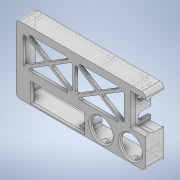
# Autodesk Inventor part: top_squr
Saved by Autodesk Inventor 2021 (Build 250183000, 183)
## iProperties
Created: 2025-01-04
Part Number: top_squr
Material: Generic
Document SubType Name: Modeling
Designer: Toby
Density: 1 g/cm^3
Appearance: Default
Author: Toby
Autodesk Inventor part; units mm, degrees
ref_plane "YZ Plane" through (0, 0, 0) normal (1, 0, 0) x (0, 1, 0)
ref_plane "XZ Plane" through (0, 0, 0) normal (0, 1, 0) x (-1, 0, 0)
ref_plane "XY Plane" through (0, 0, 0) normal (0, 0, 1) x (1, 0, 0)
sketch "Sketch1" plane through (0, 0, 0) normal (0, 0, 1) x (1, 0, 0)
  line L0 (-50, 26) -> (50, 26)
  line L1 (50, 26) -> (50, -26)
  line L2 (50, -26) -> (-50, -26)
  line L3 (-50, -26) -> (-50, 26)
  point P0 (0, 0)
  dimension "d0" = 100
  dimension "d1" = 52
  dimension "d2" = 26
  dimension "d3" = 50
  constraints: 8 end point, 2 parallel, 1 horizontal, 1 perpendicular
  measures "d0" distance of L0.start L0.end
  measures "d1" distance of L2.end L0.start
  measures "d2" distance from line of point (0, 0) L0
  measures "d3" distance from line of point (0, 0) L3
extrude "Extrusion1" add sketch "Sketch1" along normal blind 2
sketch "Sketch2" plane through (0, 0, 0) normal (0, 0, -1) x (-1, 0, 0)
  line L0 (-50, -26) -> (-50, 26) projected
  line L1 (50, 26) -> (50, -26) projected
  line L2 (-50, 26) -> (50, 26)
  line L3 (50, 26) -> (50, -26)
  line L4 (50, -26) -> (-50, -26)
  line L5 (-50, -26) -> (-50, 26)
  line L6 (-48, 24) -> (48, 24)
  line L7 (48, 24) -> (48, -24)
  line L8 (48, -24) -> (-48, -24)
  line L9 (-48, -24) -> (-48, 24)
  point P0 (0, 0)
  dimension "d6" = 2
  dimension "d7" = 2
  dimension "d8" = 2
  dimension "d9" = 2
  constraints: 16 end point, 4 parallel, 2 horizontal, 2 perpendicular
  measures "d6" distance between parallel lines of L6 L2
  measures "d7" distance between parallel lines of L0 L9
  measures "d8" distance between parallel lines of L4 L8
  measures "d9" distance between parallel lines of L1 L7
extrude "Extrusion2" add sketch "Sketch2" along normal blind 12
sketch "Sketch3" plane through (0, 0, 2) normal (0, 0, 1) x (1, 0, 0)
  line L0 (-50, 26) -> (-50, -26) projected
  line L1 (-50, -26) -> (50, -26) projected
  circle A0 centre (15.5, -15.6) radius 8.5
  circle A1 centre (38.25, -15.6) radius 8.5
  point P0 (0, 0)
  dimension "d12" = 65.5
  dimension "d13" = 10.4
  dimension "d14" = 88.25
  dimension "d15" = 10.4
  dimension "d16" = 17
  dimension "d17" = 17
  constraints: 2 centre point, 2 coincident
  measures "d12" distance from line of L0 point (15.5, -15.6)
  measures "d13" distance from line of L1 point (15.5, -15.6)
  measures "d14" distance from line of L0 point (38.25, -15.6)
  measures "d15" distance from line of L1 point (38.25, -15.6)
  measures "d16" diameter of A0
  measures "d17" diameter of A1
extrude "Extrusion3" cut sketch "Sketch3" against normal blind 2
sketch "Sketch4" plane through (0, 0, 2) normal (0, 0, 1) x (1, 0, 0)
  line L0 (-38, -11) -> (2, -11)
  line L1 (2, -11) -> (2, -24)
  line L2 (2, -24) -> (-38, -24)
  line L3 (-38, -24) -> (-38, -11)
  line L4 (-50, -26) -> (50, -26) projected
  line L5 (-50, 26) -> (-50, -26) projected
  point P0 (0, 0)
  dimension "d20" = 40
  dimension "d21" = 13
  dimension "d22" = 2
  dimension "d23" = 12
  constraints: 8 end point, 2 parallel, 1 horizontal, 1 perpendicular
  measures "d20" distance of L0.start L0.end
  measures "d21" distance of L2.end L0.start
  measures "d22" distance between parallel lines of L4 L2
  measures "d23" distance between parallel lines of L5 L3
extrude "Extrusion4" cut sketch "Sketch4" against normal blind 2
fillet "Fillet1" radius 3 8 edges at (-48, 24, -6) (-50, 26, -5) (50, 26, -5) (48, 24, -6) (48, -24, -6) (50, -26, -5) (-50, -26, -5) (-48, -24, -6)
chamfer "Chamfer1" distance 1 angle 45 6 edges at (-18, -11, 2) (-38, -17.5, 2) (-18, -24, 2) (2, -17.5, 2) (7, -15.6, 2) (29.75, -15.6, 2)
sketch "Sketch5" plane through (0, 0, 2) normal (0, 0, 1) x (1, 0, 0)
  line L0 (50, -23) -> (50, 23) projected
  line L1 (-47, 26) -> (47, 26) projected
  line L2 (50, -3) -> (38, -3)
  line L3 (38, -3) -> (38, 26)
  line L4 (38, 26) -> (50, 26)
  line L5 (50, 26) -> (50, -3)
  line L6 (-50, 23) -> (-50, -23) projected
  line L7 (-47, -26) -> (47, -26) projected
  point P0 (0, 0)
  point P1 (47, 26)
  dimension "d30" = 88
  dimension "d31" = 29
  dimension "d32" = 23
  constraints: 8 end point, 2 parallel, 2 point on line, 1 horizontal, 1 perpendicular
  measures "d30" distance between parallel lines of L6 L3
  measures "d31" distance between parallel lines of L1 L2
  measures "d32" distance between parallel lines of L7 L2
extrude "Extrusion5" cut sketch "Sketch5" against normal blind 20
sketch "Sketch6" plane through (38, -3, 2) normal (0, 1, 0) x (1, 0, 0)
  line L0 (12, 14) -> (12, 0) projected
  line L1 (-9.25, 0) -> (9.75, 0) projected
  line L2 (12, 14) -> (0, 14)
  line L3 (0, 14) -> (0, 0)
  line L4 (0, 0) -> (12, 0)
  line L5 (12, 0) -> (12, 14)
  line L6 (0, 0) -> (0, 14) projected
  point P0 (-38, 2)
  point P1 (12, 0)
  constraints: 8 end point, 2 parallel, 1 collinear, 1 horizontal, 1 perpendicular, 1 point on line
extrude "Extrusion6" add sketch "Sketch6" along normal blind 2
sketch "Sketch7" plane through (38, 24, -12) normal (1, 0, 0) x (0, 0, -1)
  line L0 (0, -27) -> (-12, -27) projected
  line L1 (-14, -1) -> (-14, 2) projected
  line L2 (0, -27) -> (-14, -27)
  line L3 (-14, -27) -> (-14, 2)
  line L4 (-14, 2) -> (0, 2)
  line L5 (0, 2) -> (0, -27)
  point P0 (-12, -24)
  constraints: 8 end point, 2 parallel, 1 horizontal, 1 perpendicular
extrude "Extrusion7" add sketch "Sketch7" along normal blind 2
sketch "Sketch8" plane through (40, 24, -12) normal (1, 0, 0) x (0, 0, -1)
  circle A0 centre (-7, -8) radius 5.5
  circle A1 centre (-7, -21) radius 5.5
  line L0 (-14, -50) -> (0, -50) projected
  line L1 (0, -25) -> (0, 2) projected
  circle A2 centre (-7, -21) radius 2.9
  circle A3 centre (-7, -8) radius 2.9
  line L2 (0, -47) -> (0, -1) projected
  line L3 (-7, -23.9) -> (0, -23.9)
  line L4 (0, -23.9) -> (0, -18.1)
  line L5 (0, -18.1) -> (-7, -18.1)
  line L6 (-7, -18.1) -> (-7, -23.9)
  line L7 (-7, -10.9) -> (0, -10.9)
  line L8 (0, -10.9) -> (0, -5.1)
  line L9 (0, -5.1) -> (-7, -5.1)
  line L10 (-7, -5.1) -> (-7, -10.9)
  point P0 (-12, -24)
  point P1 (-7, -5.1)
  point P2 (0, -10.9)
  point P3 (0, -23.9)
  point P4 (0, -18.1)
  point P5 (-7, -18.1)
  point P6 (-2.3267, -5.1)
  point P7 (-2.3267, -10.9)
  point P8 (-2.3267, -18.1)
  point P9 (-2.3267, -23.9)
  point P10 (-7, -5.1)
  dimension "d45" = 5.8
  dimension "d46" = 5.8
  dimension "d39" = 11
  dimension "d40" = 11
  dimension "d41" = 42
  dimension "d42" = 29
  dimension "d43" = 7
  dimension "d44" = 0
  dimension "d107" = 7
  dimension "d108" = 5.8
  dimension "d109" = 5.8
  constraints: 16 end point, 4 parallel, 3 point on line, 2 centre point, 2 coincident, 2 horizontal, 2 perpendicular, 6 other
  measures "d39" diameter of A0
  measures "d40" diameter of A1
  measures "d41" distance from line of L0 A0.centre
  measures "d42" distance from line of L0 A1.centre
  measures "d43" distance from line of L1 A1.centre
  measures "d44" horizontal distance of A1.centre A0.centre
  measures "d107" distance between parallel lines of L1 L6
  measures "d108" distance between parallel lines of L5 L3
  measures "d109" distance between parallel lines of L9 L7
extrude "Extrusion8" cut sketch "Sketch8" against normal blind 2 contours A0 L7 A3 L9 | A0 L9 L1 L7 | L10 A3 | A3 L10 | A1 L3 A2 L5 | A1 L5 L1 L3 | L6 A2 | A2 L6 picked at (-2.398, -8.3375) picked at (-2.398, -21.3375)
sketch "Sketch9" plane through (40, 24, -12) normal (1, 0, 0) x (0, 0, -1)
  arc A0 (-7, -18.1) -> (-7, -23.9) centre (-7, -21) ccw projected
  circle A1 centre (-7, -21) radius 6
  point P0 (-12, -24)
  dimension "d49" = 12
  constraints: 1 centre point, 1 coincident
  measures "d49" diameter of A1
extrude "Extrusion9" cut sketch "Sketch9" along normal blind 20
chamfer "Chamfer2" distance 2 angle 45 2 edges at (45, -1, 2) (40, 12.5, 2)
sketch "Sketch10" plane through (-50, -23, 2) normal (-1, 0, 0) x (0, 0, 1)
  line L0 (-14, 41.9) -> (-14, 23.1) projected
  line L1 (-14, 37) -> (-10.5, 37)
  line L2 (-10.5, 37) -> (-10.5, 27)
  line L3 (-10.5, 27) -> (-14, 27)
  line L4 (-14, 27) -> (-14, 37)
  line L5 (-14, 22) -> (-14, 0) projected
  line L6 (-14, 11) -> (-10.5, 11)
  line L7 (-10.5, 11) -> (-10.5, 3)
  line L8 (-10.5, 3) -> (-14, 3)
  line L9 (-14, 3) -> (-14, 11)
  line L10 (-14, -3) -> (0, -3) projected
  line L11 (-10.5, 11) -> (-14, 11)
  line L12 (-14, 11) -> (-14, 13)
  line L13 (-14, 13) -> (-10.5, 13)
  line L14 (-10.5, 13) -> (-10.5, 11)
  point P0 (-2, 23)
  point P1 (-14, 44)
  dimension "d56" = 30
  dimension "d57" = 40
  dimension "d58" = 3.5
  dimension "d59" = 6
  dimension "d60" = 14
  dimension "d61" = 16
  constraints: 24 end point, 6 parallel, 3 horizontal, 3 perpendicular, 3 point on line, 1 midpoint
  measures "d56" distance between parallel lines of L10 L3
  measures "d57" distance between parallel lines of L10 L1
  measures "d58" distance between parallel lines of L4 L2
  measures "d59" distance between parallel lines of L10 L8
  measures "d60" distance between parallel lines of L10 L6
  measures "d61" distance between parallel lines of L10 L13
extrude "Extrusion10" cut sketch "Sketch10" against normal blind 2
fillet "Fillet3" radius 1 4 edges at (-49, 14, -8.5) (-49, 4, -8.5) (-49, -10, -8.5) (-49, -20, -8.5)
chamfer "Chamfer3" distance 1 angle 45 13 edges at (-47.1213, -23.1213, -12) (-48, -20.5, -12) (0, -24, -12) (47.1213, -23.1213, -12) (48, -12, -12) (-3.5, 24, -12) (-47.1213, 23.1213, -12) (-48, 17.5, -12) (38, -1.45, -12) (38, 21.45, -12) (38, 9.5, -12) (-48, -3, -12) (43, -3, -12)
sketch "Sketch11" plane through (0, 0, -12) normal (0, 0, -1) x (-1, 0, 0)
  line L0 (50, 14) -> (50, 23) projected
  line L1 (-47, -26) -> (47, -26) projected
  circle A0 centre (-35, 23) radius 1
  circle A1 centre (-10, 23) radius 1
  circle A2 centre (47, 23) radius 1
  circle A3 centre (47, 23) radius 2.5
  circle A4 centre (-10, 23) radius 2.5
  circle A5 centre (-35, 23) radius 2.5
  point P0 (0, 0)
  dimension "d68" = 3
  dimension "d69" = 49
  dimension "d70" = 60
  dimension "d71" = 49
  dimension "d72" = 85
  dimension "d73" = 49
  dimension "d74" = 2
  dimension "d75" = 2
  dimension "d76" = 2
  dimension "d77" = 5
  dimension "d78" = 5
  dimension "d79" = 5
  constraints: 6 centre point, 6 coincident
  measures "d68" distance from line of L0 point (47, 23)
  measures "d69" distance from line of L1 point (47, 23)
  measures "d70" distance from line of L0 point (-10, 23)
  measures "d71" distance from line of L1 point (-10, 23)
  measures "d72" distance from line of L0 point (-35, 23)
  measures "d73" distance from line of L1 point (-35, 23)
  measures "d74" diameter of A0
  measures "d75" diameter of A1
  measures "d76" diameter of A2
  measures "d77" diameter of A3
  measures "d78" diameter of A4
  measures "d79" diameter of A5
extrude "Extrusion11" add sketch "Sketch11" against normal blind 12
sketch "Sketch12" plane through (0, 0, -12) normal (0, 0, -1) x (-1, 0, 0)
  line L0 (50, -23) -> (50, -20) projected
  line L1 (-47, -26) -> (47, -26) projected
  circle A0 centre (47, -23) radius 1
  circle A1 centre (47, -23) radius 2.5
  point P0 (0, 0)
  dimension "d82" = 3
  dimension "d83" = 3
  dimension "d84" = 2
  dimension "d85" = 5
  constraints: 2 centre point, 2 coincident
  measures "d82" distance from line of L0 point (47, -23)
  measures "d83" distance from line of L1 point (47, -23)
  measures "d84" diameter of A0
  measures "d85" diameter of A1
extrude "Extrusion12" add sketch "Sketch12" against normal blind 12
sketch "Sketch13" plane through (0, 0, -12) normal (0, 0, -1) x (-1, 0, 0)
  arc A0 (46.2929, 23.7071) -> (47.7071, 22.2929) centre (47, 23) ccw projected
  arc A1 (47.7071, -22.2929) -> (46.2929, -23.7071) centre (47, -23) ccw projected
  point P0 (0, 0)
  constraints: 2 coincident
hole "Hole1" at (-47, 23, -12) at (-47, -23, -12) direction (0, 0, 1) diameter 2 depth 6.5 tip angle 118
sketch "Sketch14" plane through (0, 0, 0) normal (0, 0, -1) x (-1, 0, 0)
  line L0 (-47, -26) -> (47, -26) projected
  line L1 (50, -11) -> (50, -19) projected
  circle A0 centre (-47, -18) radius 2.1
  point P0 (0, 0)
  dimension "d95" = 8
  dimension "d96" = 97
  dimension "d97" = 4.2
  constraints: 1 centre point, 1 coincident
  measures "d95" distance from line of L0 point (-47, -18)
  measures "d96" distance from line of L1 point (-47, -18)
  measures "d97" diameter of A0
extrude "Extrusion13" add sketch "Sketch14" along normal blind 12
sketch "Sketch15" plane through (0, 0, -12) normal (0, 0, -1) x (-1, 0, 0)
  arc A0 (-48, -19.8466) -> (-48, -16.1534) centre (-47, -18) ccw projected
  point P0 (0, 0)
  constraints: 1 coincident
hole "Hole2" at (47, -18, -12) direction (0, 0, 1) diameter 2 depth 6.5 tip angle 118
sketch "Sketch16" plane through (0, 0, 0) normal (0, 0, -1) x (-1, 0, 0)
  line L0 (-48, -16.1534) -> (-48, -3) projected
  line L1 (-48, -3) -> (-38, -3)
  line L2 (-38, -3) -> (-38, -5)
  line L3 (-38, -5) -> (-48, -5)
  line L4 (-48, -5) -> (-48, -3)
  line L5 (-38, -3) -> (-38, 0.1) projected
  point P0 (0, 0)
  dimension "d110" = 2
  constraints: 8 end point, 2 parallel, 1 collinear, 1 horizontal, 1 perpendicular
  measures "d110" distance between parallel lines of L1 L3
extrude "Extrusion14" add sketch "Sketch16" along normal blind 11
sketch "Sketch17" plane through (0, 0, -12) normal (0, 0, -1) x (-1, 0, 0)
  line L0 (-38, 24) -> (-38, -5) projected
  line L1 (-49, -2) -> (-49, -17.3597) projected
  line L2 (-38, -1) -> (-49, -1)
  line L3 (-49, -1) -> (-49, -5)
  line L4 (-49, -5) -> (-38, -5)
  line L5 (-38, -5) -> (-38, -1)
  line L6 (-50, -1) -> (-40, -1) projected
  line L7 (-48, -5) -> (-38, -5) projected
  point P0 (0, 0)
  point P1 (-38, 21)
  point P2 (-38, -5)
  constraints: 8 end point, 2 collinear, 2 parallel, 2 point on line, 1 horizontal, 1 perpendicular
extrude "Extrusion15" add sketch "Sketch17" against normal blind 1
sketch "Sketch18" plane through (50, -23, 2) normal (1, 0, 0) x (0, 0, -1)
  line L0 (14, 22) -> (11.4721, 22) projected
  arc A0 (2.5279, 22) -> (11.4721, 22) centre (7, 26) ccw projected
  line L1 (14, 22) -> (7, 22)
  line L2 (7, 22) -> (7, 20)
  line L3 (7, 20) -> (14, 20)
  line L4 (14, 20) -> (14, 22)
  point P0 (2, 23)
  dimension "d115" = 2
  constraints: 8 end point, 2 parallel, 1 horizontal, 1 perpendicular, 1 point on circle
  measures "d115" distance of L1.end L2.end
extrude "Extrusion16" cut sketch "Sketch18" against normal blind 10
sketch "Sketch19" plane through (0, 0, -12) normal (0, 0, -1) x (-1, 0, 0)
  line L0 (-38, -5) -> (-38, -1) projected
  line L1 (-38, -5) -> (-49, -5)
  line L2 (-49, -5) -> (-49, -3)
  line L3 (-49, -3) -> (-38, -3)
  line L4 (-38, -3) -> (-38, -5)
  line L5 (-49, -5) -> (-49, -17.3597) projected
  line L6 (-40, -3) -> (-50, -3) projected
  point P0 (0, 0)
  dimension "d118" = 0
  constraints: 8 end point, 2 parallel, 1 collinear, 1 horizontal, 1 perpendicular
  measures "d118" distance between parallel lines of L3 L6
extrude "Extrusion17" cut sketch "Sketch19" against normal blind 1
fillet "Fillet4" radius 2 1 edges at (38, 9.5, 0)
sketch "Sketch23" plane through (0, 0, 0) normal (0, 0, -1) x (-1, 0, 0)
  line L0 (-39, 13.1) -> (-39, 5.9) projected
  line L1 (-39, 8.5) -> (-34, 8.5)
  line L2 (-34, 8.5) -> (-34, 10.5)
  line L3 (-34, 10.5) -> (-39, 10.5)
  line L4 (-39, 10.5) -> (-39, 8.5)
  point P0 (0, 0)
  point P1 (-39, 9.5)
  dimension "d161" = 5
  dimension "d162" = 1
  dimension "d163" = 1
  constraints: 8 end point, 2 parallel, 1 horizontal, 1 midpoint, 1 perpendicular, 1 point on line
  measures "d161" distance from line of L1.start L2
  measures "d162" distance from line of point (-39, 9.5) L1
  measures "d163" distance from line of L3 point (-39, 9.5)
extrude "Extrusion21" add sketch "Sketch23" along normal blind 11
chamfer "Chamfer6" distance 4 angle 45 1 edges at (34, 9.5, -11)
sketch "Sketch24" plane through (0, 0, 2) normal (0, 0, 1) x (1, 0, 0)
  line L0 (38, 26) -> (38, -3) projected
  line L1 (38, 26) -> (50, 26)
  line L2 (50, 26) -> (50, 19)
  line L3 (50, 19) -> (38, 19)
  line L4 (38, 19) -> (38, 26)
  line L5 (50, -23) -> (50, -3) projected
  point P0 (0, 0)
  dimension "d169" = 7
  constraints: 8 end point, 2 parallel, 1 collinear, 1 horizontal, 1 perpendicular
  measures "d169" distance between parallel lines of L3 L1
extrude "Extrusion22" add sketch "Sketch24" against normal blind 14
sketch "Sketch25" plane through (50, 19, 2) normal (1, 0, 0) x (0, 0, -1)
  arc A0 (7, -0.1) -> (7, -5.9) centre (7, -3) ccw projected
  arc A1 (7, -13.1) -> (7, -18.9) centre (7, -16) ccw projected
  circle A2 centre (7, -3) radius 6
  line L0 (2, 3) -> (14, 3) projected
  line L1 (7, -0.1) -> (14, -0.1) projected
  line L2 (8, 3) -> (14, 3)
  line L3 (14, 3) -> (14, -0.1)
  line L4 (14, -0.1) -> (8, -0.1)
  line L5 (8, -0.1) -> (8, 3)
  point P0 (2, -19)
  point P1 (12.2526, -0.1)
  point P2 (7, 3)
  dimension "d172" = 12
  constraints: 8 end point, 3 coincident, 2 parallel, 1 centre point, 1 horizontal, 1 midpoint, 1 perpendicular
  measures "d172" diameter of A2
extrude "Extrusion23" cut sketch "Sketch25" against normal blind 10
sketch "Sketch27" plane through (50, 19, 2) normal (1, 0, 0) x (0, 0, -1)
  line L0 (0, 4) -> (0, -42) projected
  line L1 (0, 1) -> (7, 1)
  line L2 (7, 1) -> (7, -3)
  line L3 (7, -3) -> (0, -3)
  line L4 (0, -3) -> (0, 1)
  arc A0 (7, -0.1) -> (7, -5.9) centre (7, -3) ccw projected
  point P0 (2, -19)
  point P1 (4.1, -3)
  point P2 (7, -0.1)
  point P3 (0, -3)
  dimension "d182" = 4
  dimension "d183" = 0
  dimension "d184" = 0
  constraints: 8 end point, 2 parallel, 1 coincident, 1 horizontal, 1 perpendicular, 1 point on line
  measures "d182" distance from line of A0.centre L1
  measures "d183" distance from line of L3 A0.centre
  measures "d184" distance from line of A0.centre L2
extrude "Extrusion24" cut sketch "Sketch27" against normal blind 10 contours L1 L2 A0 L3 L0
chamfer "Chamfer8" distance 2 angle 45 1 edges at (40, 19.5, 2)
chamfer "Chamfer9" distance 2 angle 45 2 edges at (39, 20, 2) (45, 20, 2)
fillet "Fillet5" radius 3 1 edges at (50, 26, -5)
sketch "Sketch28" plane through (0, 0, 2) normal (0, 0, 1) x (1, 0, 0)
  circle A0 centre (15.5, -15.6) radius 8.5 projected
  circle A1 centre (15.5, -15.6) radius 8.5
  circle A2 centre (38.25, -15.6) radius 8.5 projected
  circle A3 centre (38.25, -15.6) radius 8.5
  point P0 (0, 0)
  dimension "d194" = 17
  dimension "d195" = 17
  constraints: 2 centre point, 2 coincident
  measures "d194" diameter of A1
  measures "d195" diameter of A3
extrude "Extrusion25" cut sketch "Sketch28" against normal blind 5
fillet "Fillet6" radius 2 2 edges at (48, -16.1534, -5.5) (48, -19.8466, -5.5)
chamfer "Chamfer11" distance 1.5 angle 45 1 edges at (46.452, -17.8311, -3)
sketch "Sketch29" plane through (0, 0, -12) normal (0, 0, -1) x (-1, 0, 0)
  line L0 (50, -11) -> (50, -19) projected
  line L1 (-47, -26) -> (47, -26) projected
  circle A0 centre (0, -23) radius 2.5
  point P0 (0, 0)
  dimension "d205" = 50
  dimension "d206" = 3
  dimension "d207" = 5
  constraints: 1 centre point, 1 coincident
  measures "d205" distance from line of L0 point (0, -23)
  measures "d206" distance from line of L1 point (0, -23)
  measures "d207" diameter of A0
extrude "Extrusion26" add sketch "Sketch29" against normal blind 7.5
sketch "Sketch30" plane through (0, 0, -12) normal (0, 0, -1) x (-1, 0, 0)
  arc A0 (1.5, -25) -> (-1.5, -25) centre (0, -23) ccw projected
  point P0 (0, 0)
  constraints: 1 coincident
hole "Hole3" at (0, -23, -12) direction (0, 0, 1) diameter 2 depth 6.5 tip angle 118
chamfer "Chamfer12" distance 3.49 angle 45 1 edges at (0, -24, -4.5)
fillet "Fillet7" radius 2 4 edges at (2.2913, -24, -2.755) (2.2913, -24, -7.75) (-2.2913, -24, -2.755) (-2.2913, -24, -7.75)
sketch "Sketch31" plane through (0, 0, 2) normal (0, 0, 1) x (1, 0, 0)
  line L0 (-44.5, 20.5) -> (33.5, 20.5)
  line L1 (33.5, 20.5) -> (33.5, -3.5)
  line L2 (33.5, -3.5) -> (-44.5, -3.5)
  line L3 (-44.5, -3.5) -> (-44.5, 20.5)
  line L4 (47, 26) -> (-47, 26) projected
  line L5 (-50, 23) -> (-50, -23) projected
  line L6 (40, -1) -> (40, 20) projected
  point P0 (0, 0)
  dimension "d221" = 5.5
  dimension "d222" = 5.5
  dimension "d223" = 6.5
  dimension "d224" = 24
  constraints: 8 end point, 2 parallel, 1 horizontal, 1 perpendicular
  measures "d221" distance between parallel lines of L0 L4
  measures "d222" distance between parallel lines of L5 L3
  measures "d223" distance between parallel lines of L6 L1
  measures "d224" distance between parallel lines of L0 L2
extrude "Extrusion27" cut sketch "Sketch31" against normal blind 2
sketch "Sketch32" plane through (0, 0, 2) normal (0, 0, 1) x (1, 0, 0)
  line L0 (10, 20.5) -> (-44.5, 20.5) projected
  line L1 (-44.5, 20.5) -> (-5.5, -3.5) construction
  line L2 (33.5, -3.5) -> (-44.5, -3.5) projected
  line L3 (-45.0241, 19.6483) -> (-6.0241, -4.3517)
  line L4 (-4.9759, -2.6483) -> (-43.9759, 21.3517)
  arc A0 (-43.9759, 21.3517) -> (-45.0241, 19.6483) centre (-44.5, 20.5) ccw
  arc A1 (-6.0241, -4.3517) -> (-4.9759, -2.6483) centre (-5.5, -3.5) ccw
  line L5 (33.5, 20.5) -> (33.5, -3.5) projected
  line L6 (-5.5, -3.5) -> (33.5, 20.5) construction
  line L7 (-4.9759, -4.3517) -> (34.0241, 19.6483)
  line L8 (32.9759, 21.3517) -> (-6.0241, -2.6483)
  arc A2 (-6.0241, -2.6483) -> (-4.9759, -4.3517) centre (-5.5, -3.5) ccw
  arc A3 (34.0241, 19.6483) -> (32.9759, 21.3517) centre (33.5, 20.5) ccw
  line L9 (-5.5, -3.5) -> (-5.5, 20.5) construction
  line L10 (-4.5, -3.5) -> (-4.5, 20.5)
  line L11 (-6.5, 20.5) -> (-6.5, -3.5)
  arc A4 (-6.5, -3.5) -> (-4.5, -3.5) centre (-5.5, -3.5) ccw
  arc A5 (-4.5, 20.5) -> (-6.5, 20.5) centre (-5.5, 20.5) ccw
  line L12 (-5.5, 20.5) -> (-44.5, -3.5) construction
  line L13 (-6.0241, 21.3517) -> (-45.0241, -2.6483)
  line L14 (-43.9759, -4.3517) -> (-4.9759, 19.6483)
  arc A6 (-4.9759, 19.6483) -> (-6.0241, 21.3517) centre (-5.5, 20.5) ccw
  arc A7 (-45.0241, -2.6483) -> (-43.9759, -4.3517) centre (-44.5, -3.5) ccw
  line L15 (-5.5, 20.5) -> (33.5, -3.5) construction
  line L16 (-6.0241, 19.6483) -> (32.9759, -4.3517)
  line L17 (34.0241, -2.6483) -> (-4.9759, 21.3517)
  arc A8 (-4.9759, 21.3517) -> (-6.0241, 19.6483) centre (-5.5, 20.5) ccw
  arc A9 (32.9759, -4.3517) -> (34.0241, -2.6483) centre (33.5, -3.5) ccw
  point P0 (0, 0)
  point P1 (-25, 8.5)
  point P2 (14, 8.5)
  point P3 (-5.5, 8.5)
  point P4 (-25, 8.5)
  point P5 (14, 8.5)
  point P6 (-4.5, -1.7104)
  point P7 (-4.5, 18.7104)
  point P8 (12.092, 8.5)
  point P9 (-23.092, 8.5)
  point P10 (-6.5, 18.7104)
  point P11 (-6.5, -1.7104)
  point P12 (14, 7.3258)
  point P13 (15.908, 8.5)
  point P14 (14, 9.6742)
  point P15 (-25, 9.6742)
  point P16 (-26.908, 8.5)
  point P17 (-25, 7.3258)
  dimension "d227" = 2
  dimension "d228" = 2
  dimension "d229" = 2
  dimension "d230" = 2
  dimension "d231" = 2
  constraints: 40 end point, 20 point on circle, 20 tangent, 10 centre point, 7 parallel, 6 midpoint, 1 vertical
  measures "d227" diameter of A1
  measures "d228" diameter of A3
  measures "d229" diameter of A5
  measures "d230" diameter of A7
  measures "d231" diameter of A9
extrude "Extrusion28" add sketch "Sketch32" against normal blind 2 contours A6 L14 L16 A8 L0 | A5 L17 L0 | L0 L17 L8 L16 L10 | L0 A5 | L10 L16 L14 A6 | L11 L14 L4 L13 L0 | A8 L16 L14 L11 | L0 L13 A5 | L10 L8 L4 L11 L14 L16 | L17 L7 L16 L8 | L8 A3 L7 L17 | L10 A1 L4 L8 | L8 L16 L7 L2 L10 | L4 L13 L3 A0 | L4 L14 L3 L13 | L11 L2 L3 L14 L4 | L4 L8 A2 L11 | L17 L5 L2 L16 L7 | L4 A1 L2 A2 L8 | A1 A2 L2 | L2 L7 A1 | L3 L14 A7 L13 | A2 L3 L2 | L17 A9 L16 L2 L5
fillet "Fillet8" radius 1 11 edges at (-7.408, 20.5, 1) (-6.5, 18.7104, 1) (-42.592, 20.5, 1) (-44.5, 19.3258, 1) (-25, 9.6742, 1) (-26.908, 8.5, 1) (-25, 7.3258, 1) (-23.092, 8.5, 1) (-6.5, -1.7104, 1) (-7.408, -3.5, 1) (-42.592, -3.5, 1)
fillet "Fillet9" radius 1 12 edges at (33.5, -2.3258, 1) (31.592, -3.5, 1) (33.5, 19.3258, 1) (31.592, 20.5, 1) (15.908, 8.5, 1) (14, 7.3258, 1) (12.092, 8.5, 1) (14, 9.6742, 1) (-3.592, -3.5, 1) (-4.5, -1.7104, 1) (-4.5, 18.7104, 1) (-3.592, 20.5, 1)
body "Solid1"
